Autodesk Inventor part; units mm, degrees
(part 2 of 2)
sketch "Sketch14" plane through (0, 0, 0) normal (-1, 0, 0) x (0, 0, 1)
  line L0 (-8.6895, -181.1792) -> (10.5272, -181.1792) construction
  line L1 (10.5272, -181.1792) -> (10.5272, -189.9619) construction
  line L2 (10.5272, -189.9619) -> (-8.6895, -189.9619) construction
  line L3 (-8.6895, -189.9619) -> (-8.6895, -181.1792) construction
  line L4 (-17.1419, -187.5469) -> (-15.0868, -181.4509)
  line L5 (-15.0868, -181.4509) -> (-14.0889, -181.4509)
  line L6 (-14.0889, -181.4509) -> (-12.0339, -187.5469)
  line L7 (-12.0339, -187.5469) -> (-12.8885, -187.5469)
  line L8 (-12.8885, -187.5469) -> (-13.4418, -185.8426)
  line L9 (-13.4418, -185.8426) -> (-15.7686, -185.8426)
  line L10 (-15.7686, -185.8426) -> (-16.3218, -187.5469)
  line L11 (-16.3218, -187.5469) -> (-17.1419, -187.5469)
  line L12 (-13.6641, -185.151) -> (-14.6076, -182.2808)
  line L13 (-14.6076, -182.2808) -> (-15.5462, -185.151)
  line L14 (-15.5462, -185.151) -> (-13.6641, -185.151)
  line L15 (-6.7382, -187.5469) -> (-7.7904, -187.5469)
  line L16 (-7.7904, -187.5469) -> (-9.717, -185.1213)
  line L17 (-9.717, -185.1213) -> (-10.6457, -185.1213)
  line L18 (-10.6457, -185.1213) -> (-10.6457, -187.5469)
  line L19 (-10.6457, -187.5469) -> (-11.4559, -187.5469)
  line L20 (-11.4559, -187.5469) -> (-11.4559, -181.4509)
  line L21 (-11.4559, -181.4509) -> (-9.885, -181.4509)
  spline S0 degree 2 poles (-9.885, -181.4509) (-9.3613, -181.4509) (-8.6549, -181.5645) (-8.3338, -181.772) knots 0 0 0 1 2 2 2
  spline S1 degree 2 poles (-8.3338, -181.772) (-8.0127, -181.9795) (-7.6422, -182.6266) (-7.6422, -183.1058) knots 0 0 0 1 2 2 2
  spline S2 degree 2 poles (-7.6422, -183.1058) (-7.6422, -183.7727) (-8.3239, -184.6767) (-8.9068, -184.8941) knots 0 0 0 1 2 2 2
  line L22 (-8.9068, -184.8941) -> (-6.7382, -187.5469)
  spline S3 degree 2 poles (-8.4869, -183.17) (-8.4869, -182.9033) (-8.6747, -182.4932) (-8.8723, -182.3599) knots 0 0 0 1 2 2 2
  spline S4 degree 2 poles (-8.8723, -182.3599) (-9.0452, -182.2462) (-9.5046, -182.1524) (-9.8405, -182.1524) knots 0 0 0 1 2 2 2
  line L23 (-9.8405, -182.1524) -> (-10.6457, -182.1524)
  line L24 (-10.6457, -182.1524) -> (-10.6457, -184.4445)
  line L25 (-10.6457, -184.4445) -> (-9.9344, -184.4445)
  spline S5 degree 2 poles (-9.9344, -184.4445) (-9.5836, -184.4445) (-9.0254, -184.321) (-8.8327, -184.1284) knots 0 0 0 1 2 2 2
  spline S6 degree 2 poles (-8.8327, -184.1284) (-8.6549, -183.9604) (-8.4869, -183.4862) (-8.4869, -183.17) knots 0 0 0 1 2 2 2
  line L26 (-4.8313, -187.5469) -> (-4.8313, -182.1721)
  line L27 (-4.8313, -182.1721) -> (-6.8765, -182.1721)
  line L28 (-6.8765, -182.1721) -> (-6.8765, -181.4509)
  line L29 (-6.8765, -181.4509) -> (-1.976, -181.4509)
  line L30 (-1.976, -181.4509) -> (-1.976, -182.1721)
  line L31 (-1.976, -182.1721) -> (-4.0212, -182.1721)
  line L32 (-4.0212, -182.1721) -> (-4.0212, -187.5469)
  line L33 (-4.0212, -187.5469) -> (-4.8313, -187.5469)
  spline S7 degree 2 poles (0.3409, -187.6556) (-0.3211, -187.6556) (-1.2498, -187.3789) (-1.6598, -187.1813) knots 0 0 0 1 2 2 2
  line L34 (-1.6598, -187.1813) -> (-1.6598, -186.1637)
  line L35 (-1.6598, -186.1637) -> (-1.6005, -186.1637)
  spline S8 degree 2 poles (-1.6005, -186.1637) (-1.2004, -186.5391) (-0.1877, -186.9541) (0.2816, -186.9541) knots 0 0 0 1 2 2 2
  spline S9 degree 2 poles (0.2816, -186.9541) (0.9535, -186.9541) (1.6401, -186.3959) (1.6401, -185.9364) knots 0 0 0 1 2 2 2
  spline S10 degree 2 poles (1.6401, -185.9364) (1.6401, -185.5709) (1.2795, -185.1164) (0.8892, -185.0028) knots 0 0 0 1 2 2 2
  spline S11 degree 2 poles (0.8892, -185.0028) (0.6077, -184.9237) (0.1384, -184.815) (-0.2124, -184.7261) knots 0 0 0 1 2 2 2
  spline S12 degree 2 poles (-0.2124, -184.7261) (-0.5286, -184.6421) (-1.0275, -184.3902) (-1.2202, -184.1877) knots 0 0 0 1 2 2 2
  spline S13 degree 2 poles (-1.2202, -184.1877) (-1.4079, -183.9851) (-1.6154, -183.4417) (-1.6154, -183.086) knots 0 0 0 1 2 2 2
  spline S14 degree 2 poles (-1.6154, -183.086) (-1.6154, -182.345) (-0.4594, -181.3422) (0.4348, -181.3422) knots 0 0 0 1 2 2 2
  spline S15 degree 2 poles (0.4348, -181.3422) (0.9485, -181.3422) (1.8575, -181.5447) (2.2477, -181.7374) knots 0 0 0 1 2 2 2
  line L36 (2.2477, -181.7374) -> (2.2477, -182.7057)
  line L37 (2.2477, -182.7057) -> (2.1885, -182.7057)
  spline S16 degree 2 poles (2.1885, -182.7057) (1.897, -182.4389) (0.988, -182.0437) (0.4891, -182.0437) knots 0 0 0 1 2 2 2
  spline S17 degree 2 poles (0.4891, -182.0437) (-0.0741, -182.0437) (-0.7706, -182.5723) (-0.7706, -183.0021) knots 0 0 0 1 2 2 2
  spline S18 degree 2 poles (-0.7706, -183.0021) (-0.7706, -183.3874) (-0.3606, -183.8468) (0.0247, -183.9505) knots 0 0 0 1 2 2 2
  spline S19 degree 2 poles (0.0247, -183.9505) (0.2816, -184.0197) (1.0276, -184.1975) (1.2746, -184.2716) knots 0 0 0 1 2 2 2
  spline S20 degree 2 poles (1.2746, -184.2716) (1.9019, -184.4643) (2.4849, -185.2399) (2.4849, -185.808) knots 0 0 0 1 2 2 2
  spline S21 degree 2 poles (2.4849, -185.808) (2.4849, -186.1686) (2.1934, -186.8602) (1.9316, -187.1023) knots 0 0 0 1 2 2 2
  spline S22 degree 2 poles (1.9316, -187.1023) (1.6401, -187.369) (0.8991, -187.6556) (0.3409, -187.6556) knots 0 0 0 1 2 2 2
  line L38 (5.3698, -185.2498) -> (3.0629, -185.2498)
  line L39 (3.0629, -185.2498) -> (3.0629, -184.5088)
  line L40 (3.0629, -184.5088) -> (5.3698, -184.5088)
  line L41 (5.3698, -184.5088) -> (5.3698, -185.2498)
  line L42 (9.885, -187.5469) -> (6.3529, -187.5469)
  line L43 (6.3529, -187.5469) -> (6.3529, -181.4509)
  line L44 (6.3529, -181.4509) -> (7.1631, -181.4509)
  line L45 (7.1631, -181.4509) -> (7.1631, -186.8256)
  line L46 (7.1631, -186.8256) -> (9.885, -186.8256)
  line L47 (9.885, -186.8256) -> (9.885, -187.5469)
  spline S23 degree 2 poles (13.0121, -187.0628) (12.9182, -187.1319) (12.6021, -187.3789) (12.4539, -187.453) knots 0 0 0 1 2 2 2
  spline S24 degree 2 poles (12.4539, -187.453) (12.2513, -187.5617) (11.8709, -187.6753) (11.5251, -187.6753) knots 0 0 0 1 2 2 2
  spline S25 degree 2 poles (11.5251, -187.6753) (11.2435, -187.6753) (10.7347, -187.4629) (10.5421, -187.2702) knots 0 0 0 1 2 2 2
  spline S26 degree 2 poles (10.5421, -187.2702) (10.3593, -187.0825) (10.137, -186.5292) (10.137, -186.223) knots 0 0 0 1 2 2 2
  spline S27 degree 2 poles (10.137, -186.223) (10.137, -185.7487) (10.5371, -185.0769) (10.9718, -184.8842) knots 0 0 0 1 2 2 2
  spline S28 degree 2 poles (10.9718, -184.8842) (11.3572, -184.7064) (12.4045, -184.573) (13.0121, -184.5384) knots 0 0 0 1 2 2 2
  line L48 (13.0121, -184.5384) -> (13.0121, -184.3902)
  spline S29 degree 2 poles (13.0121, -184.3902) (13.0121, -184.1234) (12.8491, -183.7925) (12.7009, -183.6986) knots 0 0 0 1 2 2 2
  spline S30 degree 2 poles (12.7009, -183.6986) (12.5527, -183.6047) (12.1278, -183.5455) (11.9006, -183.5455) knots 0 0 0 1 2 2 2
  spline S31 degree 2 poles (11.9006, -183.5455) (11.6338, -183.5455) (10.9126, -183.7035) (10.5519, -183.8567) knots 0 0 0 1 2 2 2
  line L49 (10.5519, -183.8567) -> (10.5075, -183.8567)
  line L50 (10.5075, -183.8567) -> (10.5075, -183.0712)
  spline S32 degree 2 poles (10.5075, -183.0712) (10.7199, -183.0119) (11.5152, -182.8637) (11.9055, -182.8637) knots 0 0 0 1 2 2 2
  spline S33 degree 2 poles (11.9055, -182.8637) (12.3798, -182.8637) (13.0269, -183.0119) (13.2838, -183.2046) knots 0 0 0 1 2 2 2
  spline S34 degree 2 poles (13.2838, -183.2046) (13.5357, -183.3923) (13.7827, -183.9901) (13.7827, -184.4198) knots 0 0 0 1 2 2 2
  line L51 (13.7827, -184.4198) -> (13.7827, -187.5469)
  line L52 (13.7827, -187.5469) -> (13.0121, -187.5469)
  line L53 (13.0121, -187.5469) -> (13.0121, -187.0628)
  line L54 (13.0121, -186.4206) -> (13.0121, -185.151)
  spline S35 degree 2 poles (13.0121, -185.151) (12.7354, -185.1757) (11.9006, -185.2596) (11.6387, -185.3387) knots 0 0 0 1 2 2 2
  spline S36 degree 2 poles (11.6387, -185.3387) (11.3325, -185.4326) (10.9323, -185.8228) (10.9323, -186.1686) knots 0 0 0 1 2 2 2
  spline S37 degree 2 poles (10.9323, -186.1686) (10.9323, -186.5638) (11.3769, -186.964) (11.8018, -186.964) knots 0 0 0 1 2 2 2
  spline S38 degree 2 poles (11.8018, -186.964) (12.1624, -186.964) (12.7552, -186.6527) (13.0121, -186.4206) knots 0 0 0 1 2 2 2
  spline S39 degree 2 poles (18.6981, -185.1855) (18.6981, -186.3069) (17.6112, -187.6753) (16.7912, -187.6753) knots 0 0 0 1 2 2 2
  spline S40 degree 2 poles (16.7912, -187.6753) (16.4207, -187.6753) (15.8921, -187.4925) (15.6352, -187.3345) knots 0 0 0 1 2 2 2
  line L55 (15.6352, -187.3345) -> (15.5858, -187.5469)
  line L56 (15.5858, -187.5469) -> (14.8646, -187.5469)
  line L57 (14.8646, -187.5469) -> (14.8646, -181.1792)
  line L58 (14.8646, -181.1792) -> (15.6352, -181.1792)
  line L59 (15.6352, -181.1792) -> (15.6352, -183.4516)
  spline S41 degree 2 poles (15.6352, -183.4516) (15.9267, -183.1898) (16.6035, -182.844) (17.0333, -182.844) knots 0 0 0 1 2 2 2
  spline S42 degree 2 poles (17.0333, -182.844) (17.8088, -182.844) (18.6981, -184.0839) (18.6981, -185.1855) knots 0 0 0 1 2 2 2
  spline S43 degree 2 poles (17.9027, -185.2448) (17.9027, -184.4248) (17.4038, -183.5751) (16.8505, -183.5751) knots 0 0 0 1 2 2 2
  spline S44 degree 2 poles (16.8505, -183.5751) (16.5393, -183.5751) (15.8971, -183.8715) (15.6352, -184.0987) knots 0 0 0 1 2 2 2
  line L60 (15.6352, -184.0987) -> (15.6352, -186.7219)
  spline S45 degree 2 poles (15.6352, -186.7219) (15.9267, -186.8652) (16.3762, -186.9837) (16.643, -186.9837) knots 0 0 0 1 2 2 2
  spline S46 degree 2 poles (16.643, -186.9837) (17.2309, -186.9837) (17.9027, -186.1489) (17.9027, -185.2448) knots 0 0 0 1 2 2 2
  spline S47 degree 2 poles (-14.1581, -195.6473) (-14.1581, -196.087) (-14.4397, -196.8378) (-14.6966, -197.1145) knots 0 0 0 1 2 2 2
  spline S48 degree 2 poles (-14.6966, -197.1145) (-14.9534, -197.3911) (-15.7192, -197.7122) (-16.1934, -197.7122) knots 0 0 0 1 2 2 2
  spline S49 degree 2 poles (-16.1934, -197.7122) (-16.6281, -197.7122) (-17.4778, -197.5196) (-17.789, -197.3664) knots 0 0 0 1 2 2 2
  line L61 (-17.789, -197.3664) -> (-17.789, -196.5019)
  line L62 (-17.789, -196.5019) -> (-17.7297, -196.5019)
  spline S50 degree 2 poles (-17.7297, -196.5019) (-17.6359, -196.5711) (-17.2851, -196.7489) (-17.0727, -196.828) knots 0 0 0 1 2 2 2
  spline S51 degree 2 poles (-17.0727, -196.828) (-16.8307, -196.9119) (-16.4305, -197.0058) (-16.1786, -197.0058) knots 0 0 0 1 2 2 2
  spline S52 degree 2 poles (-16.1786, -197.0058) (-15.9316, -197.0058) (-15.4672, -196.828) (-15.2992, -196.6353) knots 0 0 0 1 2 2 2
  spline S53 degree 2 poles (-15.2992, -196.6353) (-15.1461, -196.4525) (-14.988, -195.9684) (-14.988, -195.6424) knots 0 0 0 1 2 2 2
  spline S54 degree 2 poles (-14.988, -195.6424) (-14.988, -195.3163) (-15.1659, -194.9014) (-15.3338, -194.763) knots 0 0 0 1 2 2 2
  spline S55 degree 2 poles (-15.3338, -194.763) (-15.5067, -194.6099) (-16.0205, -194.4814) (-16.3317, -194.4814) knots 0 0 0 1 2 2 2
  spline S56 degree 2 poles (-16.3317, -194.4814) (-16.6676, -194.4814) (-17.3345, -194.5852) (-17.5371, -194.6296) knots 0 0 0 1 2 2 2
  line L63 (-17.5371, -194.6296) -> (-17.5371, -191.4878)
  line L64 (-17.5371, -191.4878) -> (-14.1927, -191.4878)
  line L65 (-14.1927, -191.4878) -> (-14.1927, -192.2041)
  line L66 (-14.1927, -192.2041) -> (-16.7516, -192.2041)
  line L67 (-16.7516, -192.2041) -> (-16.7516, -193.8294)
  spline S57 degree 2 poles (-16.7516, -193.8294) (-16.6034, -193.8096) (-16.3169, -193.7948) (-16.1983, -193.7948) knots 0 0 0 1 2 2 2
  spline S58 degree 2 poles (-16.1983, -193.7948) (-15.729, -193.7948) (-15.0819, -193.9479) (-14.7855, -194.1752) knots 0 0 0 1 2 2 2
  spline S59 degree 2 poles (-14.7855, -194.1752) (-14.4841, -194.4024) (-14.1581, -195.094) (-14.1581, -195.6473) knots 0 0 0 1 2 2 2
  line L68 (-10.7445, -191.2161) -> (-13.1306, -198.9077)
  line L69 (-13.1306, -198.9077) -> (-13.8222, -198.9077)
  line L70 (-13.8222, -198.9077) -> (-11.446, -191.2161)
  line L71 (-11.446, -191.2161) -> (-10.7445, -191.2161)
  line L72 (-6.3133, -197.5838) -> (-10.0727, -197.5838)
  line L73 (-10.0727, -197.5838) -> (-10.0727, -196.7193)
  spline S60 degree 2 poles (-10.0727, -196.7193) (-9.6676, -196.3389) (-8.9464, -195.6325) (-8.6006, -195.2521) knots 0 0 0 1 2 2 2
  spline S61 degree 2 poles (-8.6006, -195.2521) (-7.904, -194.4864) (-7.3952, -193.5675) (-7.3952, -193.0785) knots 0 0 0 1 2 2 2
  spline S62 degree 2 poles (-7.3952, -193.0785) (-7.3952, -192.8216) (-7.5533, -192.4363) (-7.6965, -192.3128) knots 0 0 0 1 2 2 2
  spline S63 degree 2 poles (-7.6965, -192.3128) (-7.8398, -192.1893) (-8.2152, -192.0658) (-8.4425, -192.0658) knots 0 0 0 1 2 2 2
  spline S64 degree 2 poles (-8.4425, -192.0658) (-8.6598, -192.0658) (-9.1044, -192.1745) (-9.307, -192.2584) knots 0 0 0 1 2 2 2
  spline S65 degree 2 poles (-9.307, -192.2584) (-9.4799, -192.3276) (-9.801, -192.5252) (-9.8998, -192.5944) knots 0 0 0 1 2 2 2
  line L74 (-9.8998, -192.5944) -> (-9.9443, -192.5944)
  line L75 (-9.9443, -192.5944) -> (-9.9443, -191.7249)
  spline S66 degree 2 poles (-9.9443, -191.7249) (-9.6923, -191.6014) (-8.7883, -191.3593) (-8.3832, -191.3593) knots 0 0 0 1 2 2 2
  spline S67 degree 2 poles (-8.3832, -191.3593) (-7.5286, -191.3593) (-6.5653, -192.2634) (-6.5653, -193.034) knots 0 0 0 1 2 2 2
  spline S68 degree 2 poles (-6.5653, -193.034) (-6.5653, -193.3946) (-6.7332, -193.9973) (-6.8814, -194.2542) knots 0 0 0 1 2 2 2
  spline S69 degree 2 poles (-6.8814, -194.2542) (-7.0296, -194.521) (-7.4594, -195.0446) (-7.6965, -195.2966) knots 0 0 0 1 2 2 2
  spline S70 degree 2 poles (-7.6965, -195.2966) (-8.0819, -195.7165) (-9.0254, -196.6155) (-9.307, -196.8774) knots 0 0 0 1 2 2 2
  line L76 (-9.307, -196.8774) -> (-6.3133, -196.8774)
  line L77 (-6.3133, -196.8774) -> (-6.3133, -197.5838)
  line L78 (-1.7389, -197.5838) -> (-5.4982, -197.5838)
  line L79 (-5.4982, -197.5838) -> (-5.4982, -196.7193)
  spline S71 degree 2 poles (-5.4982, -196.7193) (-5.0931, -196.3389) (-4.3719, -195.6325) (-4.0261, -195.2521) knots 0 0 0 1 2 2 2
  spline S72 degree 2 poles (-4.0261, -195.2521) (-3.3295, -194.4864) (-2.8207, -193.5675) (-2.8207, -193.0785) knots 0 0 0 1 2 2 2
  spline S73 degree 2 poles (-2.8207, -193.0785) (-2.8207, -192.8216) (-2.9788, -192.4363) (-3.1221, -192.3128) knots 0 0 0 1 2 2 2
  spline S74 degree 2 poles (-3.1221, -192.3128) (-3.2653, -192.1893) (-3.6408, -192.0658) (-3.868, -192.0658) knots 0 0 0 1 2 2 2
  spline S75 degree 2 poles (-3.868, -192.0658) (-4.0854, -192.0658) (-4.53, -192.1745) (-4.7325, -192.2584) knots 0 0 0 1 2 2 2
  spline S76 degree 2 poles (-4.7325, -192.2584) (-4.9054, -192.3276) (-5.2265, -192.5252) (-5.3253, -192.5944) knots 0 0 0 1 2 2 2
  line L80 (-5.3253, -192.5944) -> (-5.3698, -192.5944)
  line L81 (-5.3698, -192.5944) -> (-5.3698, -191.7249)
  spline S77 degree 2 poles (-5.3698, -191.7249) (-5.1178, -191.6014) (-4.2138, -191.3593) (-3.8087, -191.3593) knots 0 0 0 1 2 2 2
  spline S78 degree 2 poles (-3.8087, -191.3593) (-2.9541, -191.3593) (-1.9908, -192.2634) (-1.9908, -193.034) knots 0 0 0 1 2 2 2
  spline S79 degree 2 poles (-1.9908, -193.034) (-1.9908, -193.3946) (-2.1588, -193.9973) (-2.307, -194.2542) knots 0 0 0 1 2 2 2
  spline S80 degree 2 poles (-2.307, -194.2542) (-2.4552, -194.521) (-2.8849, -195.0446) (-3.1221, -195.2966) knots 0 0 0 1 2 2 2
  spline S81 degree 2 poles (-3.1221, -195.2966) (-3.5074, -195.7165) (-4.4509, -196.6155) (-4.7325, -196.8774) knots 0 0 0 1 2 2 2
  line L82 (-4.7325, -196.8774) -> (-1.7389, -196.8774)
  line L83 (-1.7389, -196.8774) -> (-1.7389, -197.5838)
  line L84 (1.6105, -191.2161) -> (-0.7756, -198.9077)
  line L85 (-0.7756, -198.9077) -> (-1.4672, -198.9077)
  line L86 (-1.4672, -198.9077) -> (0.909, -191.2161)
  line L87 (0.909, -191.2161) -> (1.6105, -191.2161)
  line L88 (6.0417, -197.5838) -> (2.2823, -197.5838)
  line L89 (2.2823, -197.5838) -> (2.2823, -196.7193)
  spline S82 degree 2 poles (2.2823, -196.7193) (2.6874, -196.3389) (3.4087, -195.6325) (3.7545, -195.2521) knots 0 0 0 1 2 2 2
  spline S83 degree 2 poles (3.7545, -195.2521) (4.451, -194.4864) (4.9598, -193.5675) (4.9598, -193.0785) knots 0 0 0 1 2 2 2
  spline S84 degree 2 poles (4.9598, -193.0785) (4.9598, -192.8216) (4.8017, -192.4363) (4.6585, -192.3128) knots 0 0 0 1 2 2 2
  spline S85 degree 2 poles (4.6585, -192.3128) (4.5152, -192.1893) (4.1398, -192.0658) (3.9125, -192.0658) knots 0 0 0 1 2 2 2
  spline S86 degree 2 poles (3.9125, -192.0658) (3.6952, -192.0658) (3.2506, -192.1745) (3.048, -192.2584) knots 0 0 0 1 2 2 2
  spline S87 degree 2 poles (3.048, -192.2584) (2.8751, -192.3276) (2.554, -192.5252) (2.4552, -192.5944) knots 0 0 0 1 2 2 2
  line L90 (2.4552, -192.5944) -> (2.4108, -192.5944)
  line L91 (2.4108, -192.5944) -> (2.4108, -191.7249)
  spline S88 degree 2 poles (2.4108, -191.7249) (2.6627, -191.6014) (3.5667, -191.3593) (3.9718, -191.3593) knots 0 0 0 1 2 2 2
  spline S89 degree 2 poles (3.9718, -191.3593) (4.8264, -191.3593) (5.7898, -192.2634) (5.7898, -193.034) knots 0 0 0 1 2 2 2
  spline S90 degree 2 poles (5.7898, -193.034) (5.7898, -193.3946) (5.6218, -193.9973) (5.4736, -194.2542) knots 0 0 0 1 2 2 2
  spline S91 degree 2 poles (5.4736, -194.2542) (5.3254, -194.521) (4.8956, -195.0446) (4.6585, -195.2966) knots 0 0 0 1 2 2 2
  spline S92 degree 2 poles (4.6585, -195.2966) (4.2732, -195.7165) (3.3296, -196.6155) (3.048, -196.8774) knots 0 0 0 1 2 2 2
  line L92 (3.048, -196.8774) -> (6.0417, -196.8774)
  line L93 (6.0417, -196.8774) -> (6.0417, -197.5838)
  spline S93 degree 2 poles (10.6507, -194.5358) (10.6507, -196.1759) (9.6973, -197.7122) (8.7044, -197.7122) knots 0 0 0 1 2 2 2
  spline S94 degree 2 poles (8.7044, -197.7122) (7.6966, -197.7122) (6.7531, -196.1462) (6.7531, -194.5407) knots 0 0 0 1 2 2 2
  spline S95 degree 2 poles (6.7531, -194.5407) (6.7531, -192.8908) (7.7065, -191.3643) (8.7044, -191.3643) knots 0 0 0 1 2 2 2
  spline S96 degree 2 poles (8.7044, -191.3643) (9.7072, -191.3643) (10.6507, -192.9451) (10.6507, -194.5358) knots 0 0 0 1 2 2 2
  spline S97 degree 2 poles (9.6035, -196.3932) (9.722, -196.0919) (9.8208, -195.1632) (9.8208, -194.5358) knots 0 0 0 1 2 2 2
  spline S98 degree 2 poles (9.8208, -194.5358) (9.8208, -193.9084) (9.722, -192.9846) (9.5985, -192.6734) knots 0 0 0 1 2 2 2
  spline S99 degree 2 poles (9.5985, -192.6734) (9.475, -192.3622) (9.0452, -192.0411) (8.7044, -192.0411) knots 0 0 0 1 2 2 2
  spline S100 degree 2 poles (8.7044, -192.0411) (8.3635, -192.0411) (7.9238, -192.3622) (7.7954, -192.6833) knots 0 0 0 1 2 2 2
  spline S101 degree 2 poles (7.7954, -192.6833) (7.6719, -192.9945) (7.583, -193.943) (7.583, -194.5407) knots 0 0 0 1 2 2 2
  spline S102 degree 2 poles (7.583, -194.5407) (7.583, -195.1829) (7.662, -196.0425) (7.7905, -196.3784) knots 0 0 0 1 2 2 2
  spline S103 degree 2 poles (7.7905, -196.3784) (7.909, -196.6946) (8.3487, -197.0354) (8.7044, -197.0354) knots 0 0 0 1 2 2 2
  spline S104 degree 2 poles (8.7044, -197.0354) (9.0403, -197.0354) (9.48, -196.7143) (9.6035, -196.3932) knots 0 0 0 1 2 2 2
  line L94 (15.1906, -197.5838) -> (11.4313, -197.5838)
  line L95 (11.4313, -197.5838) -> (11.4313, -196.7193)
  spline S105 degree 2 poles (11.4313, -196.7193) (11.8363, -196.3389) (12.5576, -195.6325) (12.9034, -195.2521) knots 0 0 0 1 2 2 2
  spline S106 degree 2 poles (12.9034, -195.2521) (13.5999, -194.4864) (14.1088, -193.5675) (14.1088, -193.0785) knots 0 0 0 1 2 2 2
  spline S107 degree 2 poles (14.1088, -193.0785) (14.1088, -192.8216) (13.9507, -192.4363) (13.8074, -192.3128) knots 0 0 0 1 2 2 2
  spline S108 degree 2 poles (13.8074, -192.3128) (13.6642, -192.1893) (13.2887, -192.0658) (13.0615, -192.0658) knots 0 0 0 1 2 2 2
  spline S109 degree 2 poles (13.0615, -192.0658) (12.8441, -192.0658) (12.3995, -192.1745) (12.197, -192.2584) knots 0 0 0 1 2 2 2
  spline S110 degree 2 poles (12.197, -192.2584) (12.0241, -192.3276) (11.703, -192.5252) (11.6042, -192.5944) knots 0 0 0 1 2 2 2
  line L96 (11.6042, -192.5944) -> (11.5597, -192.5944)
  line L97 (11.5597, -192.5944) -> (11.5597, -191.7249)
  spline S111 degree 2 poles (11.5597, -191.7249) (11.8116, -191.6014) (12.7157, -191.3593) (13.1208, -191.3593) knots 0 0 0 1 2 2 2
  spline S112 degree 2 poles (13.1208, -191.3593) (13.9754, -191.3593) (14.9387, -192.2634) (14.9387, -193.034) knots 0 0 0 1 2 2 2
  spline S113 degree 2 poles (14.9387, -193.034) (14.9387, -193.3946) (14.7707, -193.9973) (14.6225, -194.2542) knots 0 0 0 1 2 2 2
  spline S114 degree 2 poles (14.6225, -194.2542) (14.4743, -194.521) (14.0445, -195.0446) (13.8074, -195.2966) knots 0 0 0 1 2 2 2
  spline S115 degree 2 poles (13.8074, -195.2966) (13.4221, -195.7165) (12.4786, -196.6155) (12.197, -196.8774) knots 0 0 0 1 2 2 2
  line L98 (12.197, -196.8774) -> (15.1906, -196.8774)
  line L99 (15.1906, -196.8774) -> (15.1906, -197.5838)
  spline S116 degree 2 poles (19.859, -195.6078) (19.859, -196.0771) (19.5477, -196.8724) (19.2859, -197.1392) knots 0 0 0 1 2 2 2
  spline S117 degree 2 poles (19.2859, -197.1392) (19.0142, -197.4208) (18.3325, -197.7122) (17.9225, -197.7122) knots 0 0 0 1 2 2 2
  spline S118 degree 2 poles (17.9225, -197.7122) (17.5124, -197.7122) (16.8357, -197.4356) (16.5788, -197.1589) knots 0 0 0 1 2 2 2
  spline S119 degree 2 poles (16.5788, -197.1589) (16.2626, -196.828) (15.9069, -195.7165) (15.9069, -194.9063) knots 0 0 0 1 2 2 2
  spline S120 degree 2 poles (15.9069, -194.9063) (15.9069, -194.1109) (16.233, -192.8315) (16.5738, -192.3572) knots 0 0 0 1 2 2 2
  spline S121 degree 2 poles (16.5738, -192.3572) (16.9048, -191.8929) (17.9521, -191.3742) (18.6388, -191.3742) knots 0 0 0 1 2 2 2
  spline S122 degree 2 poles (18.6388, -191.3742) (18.8413, -191.3742) (19.197, -191.4137) (19.3304, -191.4581) knots 0 0 0 1 2 2 2
  line L100 (19.3304, -191.4581) -> (19.3304, -192.2436)
  line L101 (19.3304, -192.2436) -> (19.2958, -192.2436)
  spline S123 degree 2 poles (19.2958, -192.2436) (19.1822, -192.1843) (18.7672, -192.0806) (18.5301, -192.0806) knots 0 0 0 1 2 2 2
  spline S124 degree 2 poles (18.5301, -192.0806) (17.7693, -192.0806) (16.8357, -193.1081) (16.7467, -194.1159) knots 0 0 0 1 2 2 2
  spline S125 degree 2 poles (16.7467, -194.1159) (17.0382, -193.9133) (17.6508, -193.691) (18.0163, -193.691) knots 0 0 0 1 2 2 2
  spline S126 degree 2 poles (18.0163, -193.691) (18.372, -193.691) (18.9055, -193.8343) (19.197, -194.0517) knots 0 0 0 1 2 2 2
  spline S127 degree 2 poles (19.197, -194.0517) (19.5329, -194.3036) (19.859, -195.0841) (19.859, -195.6078) knots 0 0 0 1 2 2 2
  spline S128 degree 2 poles (19.029, -195.6424) (19.029, -195.2669) (18.8314, -194.7581) (18.6141, -194.5802) knots 0 0 0 1 2 2 2
  spline S129 degree 2 poles (18.6141, -194.5802) (18.4511, -194.4518) (18.046, -194.3678) (17.8335, -194.3678) knots 0 0 0 1 2 2 2
  spline S130 degree 2 poles (17.8335, -194.3678) (17.547, -194.3678) (17.0086, -194.5407) (16.7467, -194.7037) knots 0 0 0 1 2 2 2
  spline S131 degree 2 poles (16.7467, -194.7037) (16.7418, -194.7927) (16.7319, -194.9606) (16.7319, -195.0891) knots 0 0 0 1 2 2 2
  spline S132 degree 2 poles (16.7319, -195.0891) (16.7319, -195.7214) (16.9789, -196.497) (17.1666, -196.6995) knots 0 0 0 1 2 2 2
  spline S133 degree 2 poles (17.1666, -196.6995) (17.3395, -196.8922) (17.715, -197.0453) (17.9274, -197.0453) knots 0 0 0 1 2 2 2
  spline S134 degree 2 poles (17.9274, -197.0453) (18.4214, -197.0453) (19.029, -196.3438) (19.029, -195.6424) knots 0 0 0 1 2 2 2
  point P0 (0, 0)
  constraints: 2 other
emboss "Emboss2" sketch "Sketch14" operation cut depth 2.54 direction (1, 0, 0)
sketch "Sketch15" plane through (0, -202.6081, 48.4212) normal (0, 0, 1) x (1, 0, 0)
  line L0 (20.32, 0) -> (20.32, 250.19) projected
  line L1 (13.462, 147.1168) -> (20.32, 147.1168)
  line L2 (20.32, 147.1168) -> (20.32, 155.1178)
  line L3 (20.32, 155.1178) -> (13.462, 155.1178)
  line L4 (13.462, 155.1178) -> (13.462, 147.1168)
  line L5 (20.32, 253.365) -> (0, 253.365) projected
  point P0 (0, 202.6081)
  point P1 (16.891, 155.1178)
  dimension "d78" = 8.001
  dimension "d79" = 6.858
  dimension "d83" = 106.2482
  constraints: 8 end point, 2 parallel, 1 horizontal, 1 midpoint, 1 perpendicular, 1 point on line
  measures "d78" distance of L3.end L1.start
  measures "d79" distance between parallel lines of L0 L4
  measures "d83" distance between parallel lines of L5 L1
extrude "Extrusion9" cut sketch "Sketch15" against normal blind 6.35
sketch "Sketch18" plane through (0, -205.7831, -50.0038) normal (0, -1, 0) x (1, 0, 0)
  line L0 (16.5608, 53.2892) -> (20.32, 53.2892)
  line L1 (20.32, 53.2892) -> (20.32, 63.2968)
  line L2 (20.32, 63.2968) -> (16.5608, 63.2968)
  line L3 (16.5608, 63.2968) -> (14.8082, 61.2968)
  line L4 (16.5608, 53.2892) -> (14.8082, 55.2892)
  line L5 (14.8082, 55.2892) -> (14.8082, 61.2968)
  line L6 (20.32, 98.425) -> (0, 98.425) projected
  line L7 (20.32, 95.25) -> (20.32, 0) projected
  point P0 (18.4404, 53.2892)
  dimension "d91" = 3.7592
  dimension "d92" = 2
  dimension "d93" = 2
  dimension "d94" = 6.0076
  dimension "d95" = 10.0076
  dimension "d97" = 3.7592
  dimension "d98" = 1.7526
  dimension "d99" = 0
  dimension "d102" = 45.1358
  constraints: 12 end point, 1 horizontal, 1 midpoint, 1 parallel, 1 perpendicular
  measures "d91" distance of L1.end L2.end
  measures "d92" vertical distance of L2.end L3.end
  measures "d93" vertical distance of L0.start L4.end
  measures "d94" distance of L4.end L3.end
  measures "d95" distance of L0.end L1.end
  measures "d97" distance of L0.start L0.end
  measures "d98" distance from line of L2.end L5
  measures "d99" distance between parallel lines of L7 L1
  measures "d102" distance from line of L6 point (18.44, 53.289)
extrude "Extrusion10" cut sketch "Sketch18" against normal blind 6.35
sketch "Sketch19" plane through (0, 13.9785, -4.7779) normal (-1, 0, 0) x (0, 0, 1)
  arc A0 (-41.4654, 32.4285) -> (-44.0509, 29.843) centre (-43.3209, 31.6985) ccw projected
  circle A1 centre (-43.3209, 31.6985) radius 4.5085
  arc A2 (46.2637, 32.4285) -> (48.8491, 29.843) centre (48.1191, 31.6985) ccw projected
  circle A3 centre (48.1191, 31.6985) radius 4.5085
  circle A4 centre (-43.3209, -214.6815) radius 1.9939 projected
  circle A5 centre (-43.3209, -214.6815) radius 4.5085
  arc A6 (46.2442, -215.3599) -> (48.7975, -212.8066) centre (48.1191, -214.6815) ccw projected
  circle A7 centre (48.1191, -214.6815) radius 4.5085
  circle A8 centre (-38.2409, -49.5815) radius 4.5085
  circle A9 centre (-38.2409, -49.5815) radius 1.9939 projected
  circle A10 centre (43.0391, -49.5815) radius 4.5085
  circle A11 centre (43.0391, -49.5815) radius 1.9939 projected
  point P0 (0, 0)
  dimension "d110" = 9.017
  dimension "d111" = 9.017
  dimension "d112" = 9.017
  dimension "d113" = 9.017
  dimension "d120" = 9.017
  dimension "d121" = 0
  dimension "d122" = 0
  dimension "d123" = 9.017
  dimension "d124" = 0
  dimension "d125" = 0
  constraints: 6 centre point, 4 coincident
  measures "d110" diameter of A1
  measures "d111" diameter of A3
  measures "d112" diameter of A5
  measures "d113" diameter of A7
  measures "d120" diameter of A8
  measures "d121" distance of A9.centre A8.centre
  measures "d122" distance of A9.centre A8.centre
  measures "d123" diameter of A10
  measures "d124" distance of A11.centre A10.centre
  measures "d125" distance of A11.centre A10.centre
extrude "Extrusion11" cut sketch "Sketch19" against normal blind 5 contours A1 | A3 | A4 | A5 | A7 | A8 | A9 | A10 | A11
sketch "Sketch20" plane through (0, -205.7831, -50.0038) normal (0, -1, 0) x (1, 0, 0)
  circle A0 centre (18.034, 75.425) radius 2.032
  line L0 (20.32, 98.425) -> (0, 98.425) projected
  line L1 (20.32, 95.25) -> (20.32, 63.2968) projected
  point P0 (0, 50.0038)
  dimension "d126" = 4.064
  dimension "d127" = 23
  dimension "d128" = 2.286
  constraints: 1 centre point
  measures "d126" diameter of A0
  measures "d127" distance from line of L0 A0.centre
  measures "d128" distance from line of L1 A0.centre
extrude "Extrusion12" cut sketch "Sketch20" against normal blind 13.97
sketch "Sketch21" plane through (6.35, 0, 0) normal (1, 0, 0) x (0, 0, -1)
  circle A0 centre (-38.2612, -35.6031) radius 1.9939 projected
  arc A1 (-36.9446, -43.9621) -> (-35.2132, -41.1342) centre (-38.3882, -41.1342) ccw
  line L0 (-36.9446, -43.9621) -> (-40.0971, -45.5714)
  arc A2 (-40.0971, -45.5714) -> (-41.4581, -46.9108) centre (-38.6535, -48.3993) ccw
  line L1 (-41.0534, -42.2715) -> (-41.1957, -42.6431)
  line L2 (-35.2132, -31.0115) -> (-35.2132, -41.1342)
  line L3 (-41.4581, -46.9108) -> (-42.0712, -48.0662)
  arc A3 (-35.2132, -31.0115) -> (-36.9446, -28.1837) centre (-38.3882, -31.0115) ccw
  line L4 (-36.9446, -28.1837) -> (-40.0971, -26.5743)
  arc A4 (-41.4581, -25.2349) -> (-40.0971, -26.5743) centre (-38.6535, -23.7465) ccw
  line L5 (-41.4581, -25.2349) -> (-42.0712, -24.0796)
  line L6 (-42.0712, -24.0796) -> (-42.0712, -48.0662)
  line L7 (-42.0712, 41.2319) -> (-42.0712, -47.4903) projected
  circle A5 centre (-38.2612, -35.6031) radius 1.9939
  line L8 (46.8288, 41.2319) -> (46.8288, -196.2581) projected
  line L9 (46.8288, -28.4911) -> (46.8288, -42.7151)
  line L10 (39.9708, -40.77) -> (39.9708, -30.4361)
  circle A6 centre (43.0188, -35.6031) radius 1.9939 projected
  circle A7 centre (43.0188, -35.6031) radius 1.9939
  line L11 (41.7036, -27.6076) -> (44.8532, -26.0017)
  line L12 (46.2148, -24.6629) -> (46.8288, -23.5074)
  line L13 (41.7036, -43.5986) -> (44.8532, -45.2045)
  line L14 (46.2148, -46.5432) -> (46.8288, -47.6988)
  arc A8 (41.7036, -27.6076) -> (39.9708, -30.4361) centre (43.1458, -30.4361) ccw
  arc A9 (44.8532, -26.0017) -> (46.2148, -24.6629) centre (43.411, -23.1731) ccw
  arc A10 (39.9708, -40.77) -> (41.7036, -43.5986) centre (43.1458, -40.77) ccw
  arc A11 (46.2148, -46.5432) -> (44.8532, -45.2045) centre (43.411, -48.033) ccw
  line L15 (46.8288, -23.5074) -> (46.8288, -47.6988)
  point P0 (0, 0)
  point P1 (-37.8414, -35.6031)
  point P2 (-40.9888, -46.0266)
  point P3 (-37.853, -42.7151)
  point P4 (-37.853, -28.4911)
  point P5 (-40.9888, -26.1192)
  point P6 (43.3998, -28.4911)
  point P7 (45.745, -25.547)
  point P8 (45.745, -45.6592)
  dimension "d135" = 14.224
  dimension "d136" = 2.0396
  dimension "d137" = 2.0396
  dimension "d138" = 145
  dimension "d139" = 145
  dimension "d140" = 117.044
  dimension "d141" = 117.044
  dimension "d142" = 3.175
  dimension "d143" = 6.858
  dimension "d144" = 7.112
  dimension "d146" = 3.1525
  dimension "d147" = 0
  dimension "d148" = 0
  dimension "d149" = 3.9878
  dimension "d153" = 6.858
  dimension "d154" = 2.0396
  dimension "d155" = 145
  dimension "d156" = 2.0396
  dimension "d157" = 145
  dimension "d158" = 3.175
  dimension "d159" = 3.1496
  dimension "d160" = 3.1496
  constraints: 28 end point, 16 point on circle, 16 tangent, 11 point on line, 10 centre point, 7 equal radius, 2 coincident, 1 collinear, 1 parallel, 1 vertical
  measures "d135" distance of point (-37.853, -42.715) point (-37.853, -28.491)
  measures "d136" vertical distance of point (-40.989, -26.119) L6.start
  measures "d137" vertical distance of point (-40.989, -46.027) L3.end
  measures "d138" angle of L3 L0
  measures "d139" angle of L5 L4
  measures "d140" angle of L2 L4
  measures "d141" angle of L0 L2
  measures "d142" radius of A3
  measures "d143" distance between parallel lines of L6 L2
  measures "d144" distance of point (-37.853, -28.491) point (-37.841, -35.603)
  measures "d146" horizontal distance of L4.start L4.end
  measures "d147" distance between parallel lines of L7 L6
  measures "d148" vertical distance of A0.centre point (-37.841, -35.603)
  measures "d149" diameter of A0
  measures "d153" distance between parallel lines of L10 L9
  measures "d154" vertical distance of point (45.745, -25.547) L12.end
  measures "d155" angle of L11 L12
  measures "d156" vertical distance of point (45.745, -45.659) L14.end
  measures "d157" angle of L14 L13
  measures "d158" radius of A8
  measures "d159" horizontal distance of L11.start L11.end
  measures "d160" horizontal distance of L13.start L13.end
extrude "Extrusion13" add sketch "Sketch21" along normal blind 8.89
body "Solid1"
